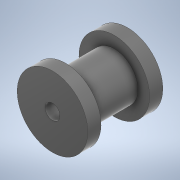
# Autodesk Inventor part: PuleyIdlerHolder
Saved by Autodesk Inventor 2020.4 (Build 244396010, 396A)
## iProperties
Created: 2020-06-05
Part Number: PuleyIdlerHolder
Material: ABS Plastic
Document SubType Name: Modeling
Designer: justi
Density: 1.06 g/cm^3
Appearance: Smooth - Black
Author: justi
Autodesk Inventor part; units mm, degrees
ref_plane "YZ Plane" through (0, 0, 0) normal (1, 0, 0) x (0, 1, 0)
ref_plane "XZ Plane" through (0, 0, 0) normal (0, 1, 0) x (-1, 0, 0)
ref_plane "XY Plane" through (0, 0, 0) normal (0, 0, 1) x (1, 0, 0)
sketch "Sketch1" plane through (0, 0, 0) normal (1, 0, 0) x (0, 1, 0)
  line L0 (0, 0) -> (-5.36, 0)
  line L1 (-5.36, 0) -> (-5.36, -11)
  line L2 (-5.36, -11) -> (0, -11)
  line L3 (0, -11) -> (0, 0)
  line L4 (0, -11) -> (-8, -11)
  line L5 (-8, -11) -> (-8, -14)
  line L6 (-8, -14) -> (0, -14)
  line L7 (0, -14) -> (0, -11)
  line L8 (0, 0) -> (-8, 0)
  line L9 (-8, 0) -> (-8, 3)
  line L10 (-8, 3) -> (0, 3)
  line L11 (0, 3) -> (0, 0)
  dimension "d0" = 5.36
  dimension "d1" = 11
  dimension "d10" = 8
  dimension "d11" = 3
  dimension "d12" = 8
  dimension "d13" = 3
  constraints: 24 end point, 6 parallel, 3 horizontal, 3 perpendicular
  measures "d0" distance of L2.end L1.end
  measures "d1" distance of L1.end L0.end
  measures "d10" distance of L6.end L5.end
  measures "d11" distance of L5.end L4.end
  measures "d12" distance of L9.end L10.end
  measures "d13" distance of L8.end L9.end
revolve "Revolution1" add sketch "Sketch1" angle 360 about axis through (0, 0, -11) along (0, 0, 1)
sketch "Sketch3" plane through (0, 0, 3) normal (0, 0, 1) x (1, 0, 0)
  point P0 (0, 0)
  point P1 (0, 0)
  constraints: 1 coincident
hole "Hole2" at (0, 0, 3) direction (0, 0, -1) diameter 3.4 end through all clearance for "Hex Head Cap Screw DIN EN 24017" size "M3" standard "DIN"
ref_plane "Work Plane1" through (0, 0, -5.5) normal (0, 0, 1) x (1, 0, 0)
body "Solid1"
